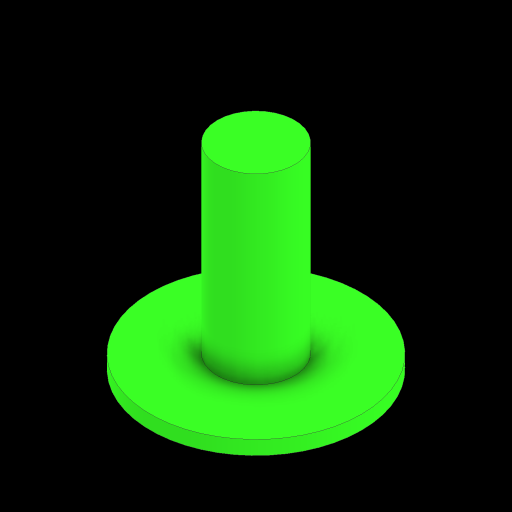
# Autodesk Inventor part: tipli
Saved by Autodesk Inventor 2023 (Build 270158000, 158)
## iProperties
Created: 2022-11-11
Part Number: tipli
Material: Generic
Document SubType Name: Modeling
Designer: gd1
Density: 1 g/cm^3
Appearance: Default
Author: gd1
Autodesk Inventor part; units mm, degrees
ref_plane "YZ Plane" through (0, 0, 0) normal (1, 0, 0) x (0, 1, 0)
ref_plane "XZ Plane" through (0, 0, 0) normal (0, 1, 0) x (-1, 0, 0)
ref_plane "XY Plane" through (0, 0, 0) normal (0, 0, 1) x (1, 0, 0)
sketch "Sketch1" plane through (0, 0, 0) normal (0, 1, 0) x (-1, 0, 0)
  circle A0 centre (0, 0) radius 7.5
  circle A1 centre (0, 0) radius 2.75
  dimension "d0" = 15
  dimension "d1" = 5.5
  constraints: 2 centre point, 2 coincident
  measures "d0" diameter of A0
  measures "d1" diameter of A1
extrude "Extrusion1" add sketch "Sketch1" along normal blind 1
extrude "Extrusion2" add sketch "Sketch1" along normal blind 14 contours A1
body "Solid1"
